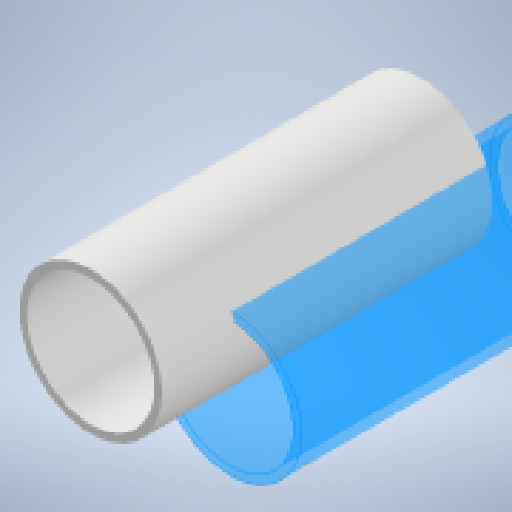
# Autodesk Inventor part: WashChamber
Saved by Autodesk Inventor 2024 (Build 280153000, 153)
## iProperties
Created: 2024-12-17
Part Number: WashChamber
Material: Generic
Document SubType Name: Modeling
Designer: Tommy Rohmann
Density: 1 g/cm^3
Appearance: Default
Author: Tommy Rohmann
Autodesk Inventor part; units mm, degrees
ref_plane "YZ Plane" through (0, 0, 0) normal (1, 0, 0) x (0, 1, 0)
ref_plane "XZ Plane" through (0, 0, 0) normal (0, 1, 0) x (-1, 0, 0)
ref_plane "XY Plane" through (0, 0, 0) normal (0, 0, 1) x (1, 0, 0)
sketch "Sketch1" plane through (0, 0, 0) normal (1, 0, 0) x (0, 1, 0)
  line L0 (-13.1213, 153.0331) -> (-13.1213, -111.8378) projected
  line L1 (-13.1213, 153.0331) -> (-19.4713, 153.0331) projected
  line L2 (-19.4713, -111.8378) -> (-19.4713, 153.0331) projected
  line L3 (-13.1213, -111.8378) -> (-19.4713, -111.8378) projected
  line L4 (-70.2713, -175.3378) -> (-70.2713, 369.4922) construction
  point P0 (0, 0)
revolve "Revolution1" add sketch "Sketch1" angle 360 about axis through (0, -70.2713, -175.3378) along (0, 0, 1)
body "Solid1"
